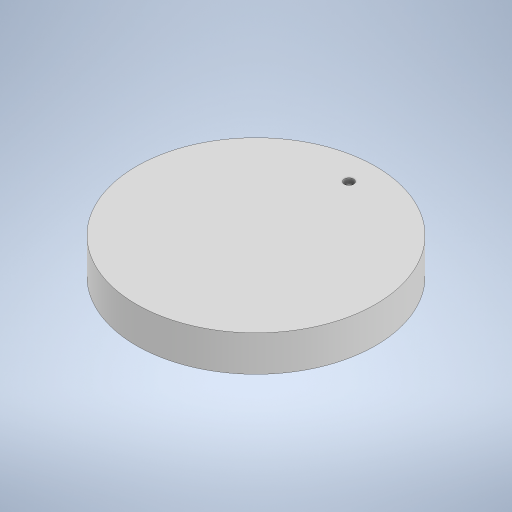
# Autodesk Inventor part: rot_no_val_th
Saved by Autodesk Inventor 2023 (Build 270158000, 158)
## iProperties
Created: 2023-05-20
Part Number: rot_no_val_th
Material: 常规
Document SubType Name: Modeling
Designer: LiuZeshu
Density: 1 g/cm^3
Appearance: 默认
Author: LiuZeshu
Autodesk Inventor part; units mm, degrees
ref_plane "YZ Plane" through (0, 0, 0) normal (1, 0, 0) x (0, 1, 0)
ref_plane "XZ Plane" through (0, 0, 0) normal (0, 1, 0) x (-1, 0, 0)
ref_plane "XY Plane" through (0, 0, 0) normal (0, 0, 1) x (1, 0, 0)
sketch "草图1" plane through (0, 0, 0) normal (0, 1, 0) x (-1, 0, 0)
  arc A0 (1.3748, -0.6) -> (-1.3748, -0.6) centre (0, 0) ccw
  line L0 (1.3748, -0.6) -> (-1.3748, -0.6)
  circle A1 centre (0, 0) radius 9
  dimension "d0" = 3
  dimension "d1" = 2.1
  dimension "d2" = 18
  constraints: 2 centre point, 2 coincident, 2 end point, 2 point on circle, 1 horizontal
  measures "d0" diameter of A0
  measures "d2" diameter of A1
extrude "拉伸1" add sketch "草图1" along normal blind 2.3
sketch "草图2" plane through (0, 2.3, 0) normal (0, 1, 0) x (1, 0, 0)
  circle A0 centre (0, 0) radius 9
  line L0 (-1.3748, 0.6) -> (1.3748, 0.6) projected
  arc A1 (-1.3748, 0.6) -> (1.3748, 0.6) centre (0, 0) ccw
  line L1 (-1.3748, 0.6) -> (1.3748, 0.6)
  dimension "d7" = 18
  constraints: 2 centre point, 2 coincident, 2 end point, 2 point on circle, 1 collinear
  measures "d7" diameter of A0
extrude "拉伸2" add sketch "草图2" along normal blind 0.4 contours A0 | L0 A1
sketch "草图5" plane through (0, 2.7, 0) normal (0, 1, 0) x (1, 0, 0)
  circle A0 centre (0, 7) radius 0.35
  line L0 (0, 7) -> (0, 0)
  dimension "d27" = 0.7
  dimension "d28" = 7
  constraints: 2 end point, 1 centre point, 1 vertical
  measures "d27" diameter of A0
  measures "d28" distance of L0.end L0.start
extrude "拉伸5" cut sketch "草图5" against normal blind 0.4
